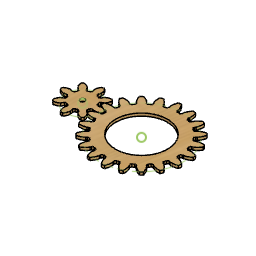
gear v4 (Autodesk Fusion 360 design; units mm, degrees)
description: Spur Gear; Module: 4.7; Num Teeth: 8; Pressure Angle: 20.0; Backlash: 0.15 mm
description: Spur Gear; Module: 4.7; Num Teeth: 20; Pressure Angle: 20.0; Backlash: 0.15 mm
Autodesk Fusion 360 part; units mm, degrees
sketch "Sketch1" plane through (0, 0, 0) normal (0, 0, 1) x (1, 0, 0) in component "Spur Gear (8 teeth)"
  circle A0 centre (0, 0) radius 13.1092
  circle A1 centre (0, 0) radius 2.55
extrude "Extrude1" add sketch "Sketch1" along normal blind 3 makes body 1 in component "Spur Gear (8 teeth)"
sketch "Sketch2" plane through (0, 0, 0) normal (0, 0, 1) x (1, 0, 0) in component "Spur Gear (8 teeth)"
  spline S0 degree 5 poles (17.2808, -3.6699) (17.2982, -3.6736) (17.3331, -3.6803) (17.3856, -3.6883) (17.4561, -3.6953) (17.5449, -3.6988) (17.6342, -3.6986) (17.7238, -3.6963) (17.8136, -3.6927) (17.9035, -3.6883) (17.9935, -3.683) (18.0835, -3.6763) (18.1738, -3.668) (18.2641, -3.6577) (18.3546, -3.6456) (18.4452, -3.6319) (18.5359, -3.6167) (18.6266, -3.6003) (18.7174, -3.5828) (18.8081, -3.5642) (18.8988, -3.5446) (18.9896, -3.5239) (19.0803, -3.5019) (19.171, -3.4788) (19.2618, -3.4545) (19.3525, -3.4291) (19.4431, -3.4026) (19.5337, -3.375) (19.6243, -3.3465) (19.7147, -3.317) (19.8052, -3.2865) (19.8955, -3.255) (19.9858, -3.2226) (20.0759, -3.1891) (20.166, -3.1547) (20.256, -3.1194) (20.3459, -3.0831) (20.4356, -3.0459) (20.5253, -3.0078) (20.6148, -2.9688) (20.7042, -2.929) (20.7935, -2.8882) (20.8826, -2.8466) (20.9716, -2.8041) (21.0604, -2.7607) (21.1491, -2.7165) (21.2376, -2.6715) (21.3259, -2.6256) (21.4141, -2.5789) (21.5021, -2.5313) (21.59, -2.483) (21.6776, -2.4338) (21.7651, -2.3839) (21.8523, -2.3331) (21.9394, -2.2816) (22.0263, -2.2292) (22.1129, -2.1761) (22.1994, -2.1223) (22.2856, -2.0676) (22.3716, -2.0122) (22.4574, -1.956) (22.543, -1.8991) (22.6283, -1.8414) (22.7134, -1.783) (22.7983, -1.7239) (22.8829, -1.664) (22.9673, -1.6034) (23.0514, -1.542) (23.1353, -1.48) (23.2189, -1.4172) (23.3022, -1.3538) (23.3687, -1.3024) (23.4184, -1.2636) (23.4515, -1.2376) (23.4681, -1.2245) knots 0 0 0 0 0 0 0.01428571 0.02857143 0.04285714 0.05714286 0.07142857 0.08571429 0.1 0.11428571 0.12857143 0.14285714 0.15714286 0.17142857 0.18571429 0.2 0.21428571 0.22857143 0.24285714 0.25714286 0.27142857 0.28571429 0.3 0.31428571 0.32857143 0.34285714 0.35714286 0.37142857 0.38571429 0.4 0.41428571 0.42857143 0.44285714 0.45714286 0.47142857 0.48571429 0.5 0.51428571 0.52857143 0.54285714 0.55714286 0.57142857 0.58571429 0.6 0.61428571 0.62857143 0.64285714 0.65714286 0.67142857 0.68571429 0.7 0.71428571 0.72857143 0.74285714 0.75714286 0.77142857 0.78571429 0.8 0.81428571 0.82857143 0.84285714 0.85714286 0.87142857 0.88571429 0.9 0.91428571 0.92857143 0.94285714 0.95714286 0.97142857 0.98571429 1 1 1 1 1 1
  spline S1 degree 5 poles (17.2808, 3.6699) (17.2982, 3.6736) (17.3331, 3.6803) (17.3856, 3.6883) (17.4561, 3.6953) (17.5449, 3.6988) (17.6342, 3.6986) (17.7238, 3.6963) (17.8136, 3.6927) (17.9035, 3.6883) (17.9935, 3.683) (18.0835, 3.6763) (18.1738, 3.668) (18.2641, 3.6577) (18.3546, 3.6456) (18.4452, 3.6319) (18.5359, 3.6167) (18.6266, 3.6003) (18.7174, 3.5828) (18.8081, 3.5642) (18.8988, 3.5446) (18.9896, 3.5239) (19.0803, 3.5019) (19.171, 3.4788) (19.2618, 3.4545) (19.3525, 3.4291) (19.4431, 3.4026) (19.5337, 3.375) (19.6243, 3.3465) (19.7147, 3.317) (19.8052, 3.2865) (19.8955, 3.255) (19.9858, 3.2226) (20.0759, 3.1891) (20.166, 3.1547) (20.256, 3.1194) (20.3459, 3.0831) (20.4356, 3.0459) (20.5253, 3.0078) (20.6148, 2.9688) (20.7042, 2.929) (20.7935, 2.8882) (20.8826, 2.8466) (20.9716, 2.8041) (21.0604, 2.7607) (21.1491, 2.7165) (21.2376, 2.6715) (21.3259, 2.6256) (21.4141, 2.5789) (21.5021, 2.5313) (21.59, 2.483) (21.6776, 2.4338) (21.7651, 2.3839) (21.8523, 2.3331) (21.9394, 2.2816) (22.0263, 2.2292) (22.1129, 2.1761) (22.1994, 2.1223) (22.2856, 2.0676) (22.3716, 2.0122) (22.4574, 1.956) (22.543, 1.8991) (22.6283, 1.8414) (22.7134, 1.783) (22.7983, 1.7239) (22.8829, 1.664) (22.9673, 1.6034) (23.0514, 1.542) (23.1353, 1.48) (23.2189, 1.4172) (23.3022, 1.3538) (23.3687, 1.3024) (23.4184, 1.2636) (23.4515, 1.2376) (23.4681, 1.2245) knots 0 0 0 0 0 0 0.01428571 0.02857143 0.04285714 0.05714286 0.07142857 0.08571429 0.1 0.11428571 0.12857143 0.14285714 0.15714286 0.17142857 0.18571429 0.2 0.21428571 0.22857143 0.24285714 0.25714286 0.27142857 0.28571429 0.3 0.31428571 0.32857143 0.34285714 0.35714286 0.37142857 0.38571429 0.4 0.41428571 0.42857143 0.44285714 0.45714286 0.47142857 0.48571429 0.5 0.51428571 0.52857143 0.54285714 0.55714286 0.57142857 0.58571429 0.6 0.61428571 0.62857143 0.64285714 0.65714286 0.67142857 0.68571429 0.7 0.71428571 0.72857143 0.74285714 0.75714286 0.77142857 0.78571429 0.8 0.81428571 0.82857143 0.84285714 0.85714286 0.87142857 0.88571429 0.9 0.91428571 0.92857143 0.94285714 0.95714286 0.97142857 0.98571429 1 1 1 1 1 1
  arc A0 (23.4681, -1.2245) -> (23.4681, 1.2245) centre (0, 0) ccw
  line L0 (12.8134, -2.7232) -> (17.2808, -3.6699)
  line L1 (12.8134, 2.7232) -> (17.2808, 3.6699)
  line L2 (12.8134, -2.7232) -> (12.8134, 2.7232)
  point P0 (17.701, -3.6967)
  point P1 (18.1316, -3.6716)
  point P2 (18.5685, -3.6106)
  point P3 (19.0101, -3.5187)
  point P4 (19.4551, -3.3987)
  point P5 (19.9024, -3.2523)
  point P6 (20.3513, -3.0806)
  point P7 (20.8007, -2.8846)
  point P8 (21.2501, -2.6648)
  point P9 (21.6985, -2.4218)
  point P10 (22.1452, -2.1559)
  point P11 (22.5895, -1.8675)
  point P12 (23.0307, -1.557)
  point P13 (17.701, 3.6967)
  point P14 (18.1316, 3.6716)
  point P15 (18.5685, 3.6106)
  point P16 (19.0101, 3.5187)
  point P17 (19.4551, 3.3987)
  point P18 (19.9024, 3.2523)
  point P19 (20.3513, 3.0806)
  point P20 (20.8007, 2.8846)
  point P21 (21.2501, 2.6648)
  point P22 (21.6985, 2.4218)
  point P23 (22.1452, 2.1559)
  point P24 (22.5895, 1.8675)
  point P25 (23.0307, 1.557)
extrude "Extrude2" add sketch "Sketch2" along normal blind 3 bodies 1 in component "Spur Gear (8 teeth)"
fillet "Fillet1" radius 1.5875 2 edges at (12.8228, -2.7252, 1.5) (12.8228, 2.7252, 1.5) on bodies 1 in component "Spur Gear (8 teeth)"
pattern_circular "C-Pattern1" count 8 over 360 about axis through (0, 0, 0) along (0, 0, 1) of "Extrude2", "Fillet1" in component "Spur Gear (8 teeth)"
sketch "Sketch3" plane through (0, 0, 0) normal (0, 0, 1) x (1, 0, 0) in component "Spur Gear (8 teeth)"
  circle A0 centre (0, 0) radius 18.8 construction
sketch "Sketch1 (2)" plane through (0, 0, 0) normal (0, 0, 1) x (1, 0, 0) in component "Spur Gear (20 teeth)"
  circle A0 centre (0, 0) radius 41.3092
  circle A1 centre (0, 0) radius 29
  dimension "d15" = 58
  measures "d15" diameter of A1
extrude "Extrude1'" add sketch "Sketch1 (2)" along normal blind 3 separate body makes body 2 in component "Spur Gear (20 teeth)"
sketch "Sketch2 (2)" plane through (0, 0, 0) normal (0, 0, 1) x (1, 0, 0) in component "Spur Gear (20 teeth)"
  spline S0 degree 5 poles (43.9761, -4.0859) (43.9984, -4.088) (44.0428, -4.0915) (44.1096, -4.095) (44.1986, -4.0963) (44.3102, -4.0933) (44.4218, -4.0869) (44.5335, -4.0786) (44.6453, -4.0691) (44.7571, -4.0588) (44.8689, -4.0478) (44.9807, -4.0357) (45.0925, -4.0223) (45.2043, -4.0072) (45.3161, -3.9904) (45.4279, -3.9722) (45.5397, -3.9527) (45.6514, -3.9322) (45.7632, -3.9107) (45.8748, -3.8884) (45.9865, -3.8651) (46.0981, -3.841) (46.2096, -3.8158) (46.3211, -3.7897) (46.4326, -3.7625) (46.544, -3.7344) (46.6553, -3.7054) (46.7666, -3.6755) (46.8778, -3.6448) (46.9889, -3.6133) (47.1, -3.581) (47.211, -3.5479) (47.3219, -3.514) (47.4328, -3.4793) (47.5436, -3.4438) (47.6543, -3.4075) (47.7649, -3.3705) (47.8754, -3.3327) (47.9858, -3.2941) (48.0962, -3.2549) (48.2064, -3.2149) (48.3166, -3.1742) (48.4266, -3.1328) (48.5366, -3.0908) (48.6465, -3.048) (48.7563, -3.0045) (48.8659, -2.9603) (48.9755, -2.9155) (49.0849, -2.87) (49.1943, -2.8239) (49.3035, -2.7771) (49.4126, -2.7296) (49.5216, -2.6815) (49.6305, -2.6328) (49.7393, -2.5834) (49.848, -2.5334) (49.9565, -2.4828) (50.0649, -2.4316) (50.1732, -2.3797) (50.2814, -2.3272) (50.3894, -2.2742) (50.4973, -2.2205) (50.6051, -2.1662) (50.7128, -2.1114) (50.8203, -2.0559) (50.9277, -1.9999) (51.035, -1.9433) (51.1421, -1.8861) (51.249, -1.8283) (51.3559, -1.77) (51.4626, -1.7111) (51.5478, -1.6635) (51.6117, -1.6276) (51.6542, -1.6035) (51.6755, -1.5915) knots 0 0 0 0 0 0 0.01428571 0.02857143 0.04285714 0.05714286 0.07142857 0.08571429 0.1 0.11428571 0.12857143 0.14285714 0.15714286 0.17142857 0.18571429 0.2 0.21428571 0.22857143 0.24285714 0.25714286 0.27142857 0.28571429 0.3 0.31428571 0.32857143 0.34285714 0.35714286 0.37142857 0.38571429 0.4 0.41428571 0.42857143 0.44285714 0.45714286 0.47142857 0.48571429 0.5 0.51428571 0.52857143 0.54285714 0.55714286 0.57142857 0.58571429 0.6 0.61428571 0.62857143 0.64285714 0.65714286 0.67142857 0.68571429 0.7 0.71428571 0.72857143 0.74285714 0.75714286 0.77142857 0.78571429 0.8 0.81428571 0.82857143 0.84285714 0.85714286 0.87142857 0.88571429 0.9 0.91428571 0.92857143 0.94285714 0.95714286 0.97142857 0.98571429 1 1 1 1 1 1
  spline S1 degree 5 poles (43.9761, 4.0859) (43.9984, 4.088) (44.0428, 4.0915) (44.1096, 4.095) (44.1986, 4.0963) (44.3102, 4.0933) (44.4218, 4.0869) (44.5335, 4.0786) (44.6453, 4.0691) (44.7571, 4.0588) (44.8689, 4.0478) (44.9807, 4.0357) (45.0925, 4.0223) (45.2043, 4.0072) (45.3161, 3.9904) (45.4279, 3.9722) (45.5397, 3.9527) (45.6514, 3.9322) (45.7632, 3.9107) (45.8748, 3.8884) (45.9865, 3.8651) (46.0981, 3.841) (46.2096, 3.8158) (46.3211, 3.7897) (46.4326, 3.7625) (46.544, 3.7344) (46.6553, 3.7054) (46.7666, 3.6755) (46.8778, 3.6448) (46.9889, 3.6133) (47.1, 3.581) (47.211, 3.5479) (47.3219, 3.514) (47.4328, 3.4793) (47.5436, 3.4438) (47.6543, 3.4075) (47.7649, 3.3705) (47.8754, 3.3327) (47.9858, 3.2941) (48.0962, 3.2549) (48.2064, 3.2149) (48.3166, 3.1742) (48.4266, 3.1328) (48.5366, 3.0908) (48.6465, 3.048) (48.7563, 3.0045) (48.8659, 2.9603) (48.9755, 2.9155) (49.0849, 2.87) (49.1943, 2.8239) (49.3035, 2.7771) (49.4126, 2.7296) (49.5216, 2.6815) (49.6305, 2.6328) (49.7393, 2.5834) (49.848, 2.5334) (49.9565, 2.4828) (50.0649, 2.4316) (50.1732, 2.3797) (50.2814, 2.3272) (50.3894, 2.2742) (50.4973, 2.2205) (50.6051, 2.1662) (50.7128, 2.1114) (50.8203, 2.0559) (50.9277, 1.9999) (51.035, 1.9433) (51.1421, 1.8861) (51.249, 1.8283) (51.3559, 1.77) (51.4626, 1.7111) (51.5478, 1.6635) (51.6117, 1.6276) (51.6542, 1.6035) (51.6755, 1.5915) knots 0 0 0 0 0 0 0.01428571 0.02857143 0.04285714 0.05714286 0.07142857 0.08571429 0.1 0.11428571 0.12857143 0.14285714 0.15714286 0.17142857 0.18571429 0.2 0.21428571 0.22857143 0.24285714 0.25714286 0.27142857 0.28571429 0.3 0.31428571 0.32857143 0.34285714 0.35714286 0.37142857 0.38571429 0.4 0.41428571 0.42857143 0.44285714 0.45714286 0.47142857 0.48571429 0.5 0.51428571 0.52857143 0.54285714 0.55714286 0.57142857 0.58571429 0.6 0.61428571 0.62857143 0.64285714 0.65714286 0.67142857 0.68571429 0.7 0.71428571 0.72857143 0.74285714 0.75714286 0.77142857 0.78571429 0.8 0.81428571 0.82857143 0.84285714 0.85714286 0.87142857 0.88571429 0.9 0.91428571 0.92857143 0.94285714 0.95714286 0.97142857 0.98571429 1 1 1 1 1 1
  arc A0 (51.6755, -1.5915) -> (51.6755, 1.5915) centre (0, 0) ccw
  line L0 (41.1221, -3.8217) -> (43.9761, -4.0859)
  line L1 (41.1221, 3.8217) -> (43.9761, 4.0859)
  line L2 (41.1221, -3.8217) -> (41.1221, 3.8217)
  point P0 (44.5172, -4.0796)
  point P1 (45.0624, -4.0256)
  point P2 (45.6102, -3.9396)
  point P3 (46.1599, -3.8269)
  point P4 (46.7109, -3.6904)
  point P5 (47.2628, -3.532)
  point P6 (47.8154, -3.3531)
  point P7 (48.3682, -3.1547)
  point P8 (48.921, -2.9377)
  point P9 (49.4735, -2.7027)
  point P10 (50.0255, -2.4501)
  point P11 (50.5767, -2.1805)
  point P12 (51.1267, -1.8941)
  point P13 (44.5172, 4.0796)
  point P14 (45.0624, 4.0256)
  point P15 (45.6102, 3.9396)
  point P16 (46.1599, 3.8269)
  point P17 (46.7109, 3.6904)
  point P18 (47.2628, 3.532)
  point P19 (47.8154, 3.3531)
  point P20 (48.3682, 3.1547)
  point P21 (48.921, 2.9377)
  point P22 (49.4735, 2.7027)
  point P23 (50.0255, 2.4501)
  point P24 (50.5767, 2.1805)
  point P25 (51.1267, 1.8941)
extrude "Extrude2'" add sketch "Sketch2 (2)" along normal blind 3 bodies 2 in component "Spur Gear (20 teeth)"
fillet "Fillet1'" radius 1.5875 2 edges at (41.132, -3.8226, 1.5) (41.132, 3.8226, 1.5) on bodies 2 in component "Spur Gear (20 teeth)"
pattern_circular "C-Pattern1'" count 20 over 360 about axis through (0, 0, 0) along (0, 0, 1) of "Extrude2'", "Fillet1'" in component "Spur Gear (20 teeth)"
sketch "Sketch3 (2)" plane through (0, 0, 0) normal (0, 0, 1) x (1, 0, 0) in component "Spur Gear (20 teeth)"
  circle A0 centre (0, 0) radius 47 construction
sketch "Sketch1 (3)" plane through (65.8, 0, 0) normal (0, 0, 1) x (0.987688, -0.156434, 0)
component "Spur Gear (8 teeth)" placed x (1, 0, 0) y (0, 1, 0) z (0, 0, 1) at (0, 0, 0)
component "Spur Gear (20 teeth)" placed x (0.987688, -0.156434, 0) y (0.156434, 0.987688, 0) z (0, 0, 1) at (65.8, 0, 0)
equation "taperAngle1 = 0.0 deg"
equation "Radius = 1.5875 mm"
equation "countU = 8"
